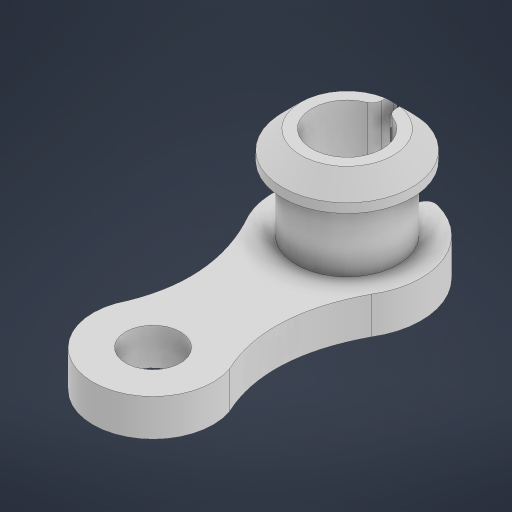
# Autodesk Inventor part: Servo_Pulley
Saved by Autodesk Inventor 2024 (Build 280153000, 153)
## iProperties
Created: 2025-09-10
Part Number: Servo_Pulley
Material: Generic
Document SubType Name: Modeling
Designer: kevin
Density: 1 g/cm^3
Appearance: Default
Author: kevin
Autodesk Inventor part; units mm, degrees
ref_plane "YZ Plane" through (0, 0, 0) normal (1, 0, 0) x (0, 1, 0)
ref_plane "XZ Plane" through (0, 0, 0) normal (0, 1, 0) x (-1, 0, 0)
ref_plane "XY Plane" through (0, 0, 0) normal (0, 0, 1) x (1, 0, 0)
sketch "Sketch1" plane through (0, 0, 0) normal (0, 1, 0) x (-1, 0, 0)
  circle A0 centre (0, 0) radius 2.95
  circle A1 centre (0, 0) radius 6.5
  circle A2 centre (0, -21) radius 8
  spline S0 degree 2 poles (6.1434, -2.1233) (2.6668, -9.5534) (7.2026, -17.5183) knots 0 0 0 1 1 1
  line L0 (0, 0) -> (0, -21) construction
  spline S1 degree 2 poles (-6.1434, -2.1233) (-2.6668, -9.5534) (-7.2026, -17.5183) knots 0 0 0 1 1 1
  point P0 (4.6554, -9.4486)
  point P1 (-4.6554, -9.4486)
  point P2 (-6.1434, -2.1233)
  point P3 (-6.812, -16.8052)
  dimension "d1" = 13
  dimension "d2" = 16
  dimension "d0" = 5.9
  dimension "d3" = 21
  constraints: 3 symmetric about line, 2 coincident, 2 end point, 1 centre point, 1 vertical, 12 other
  measures "d0" diameter of A0
  measures "d3" distance of L0.end point (0, 0)
extrude "Extrusion1" add sketch "Sketch1" along normal blind 4 contours A1 S0 S1 | A1 S0 A2 S1 | S1 A2 | A2 S0 S1
sketch "Sketch2" plane through (0, 4, 0) normal (0, 1, 0) x (1, 0, 0)
  arc A0 (6.812, 16.8052) -> (-7.2026, 17.5183) centre (0, 21) ccw projected
  arc A1 (-6.1434, 2.1233) -> (6.1434, 2.1233) centre (0, 0) ccw projected
  circle A2 centre (0, 0) radius 2.95 projected
  circle A3 centre (0, 21) radius 5.5
  line L0 (0.75, 12.2819) -> (-0.75, 12.2819)
  line L1 (-0.75, 12.2819) -> (-0.75, 29.7181)
  line L2 (-0.75, 29.7181) -> (0.75, 29.7181)
  line L3 (0.75, 29.7181) -> (0.75, 12.2819)
  line L4 (0.75, 12.2819) -> (-0.75, 29.7181) construction
  line L5 (-0.75, 12.2819) -> (0.75, 29.7181) construction
  circle A4 centre (0, 21) radius 3.8038
  point P0 (0.75, 26.4486)
  point P1 (0.75, 15.5514)
  point P2 (-0.75, 15.5514)
  point P3 (-0.75, 26.4486)
  point P4 (-0.75, 24.7291)
  point P5 (0.75, 24.7291)
  dimension "d6" = 11
  dimension "d7" = 1.5
  constraints: 12 end point, 2 centre point, 2 coincident, 2 midpoint, 2 parallel, 1 horizontal, 1 perpendicular, 2 other
  measures "d6" diameter of A3
  measures "d7" distance of L1.end L2.end
extrude "Extrusion2" cut sketch "Sketch2" against normal blind 5 contours L3 A3 L1 A0 | A0 L1 L2 L3 | L3 A4 L1 A3 | A4 L3 | L3 A4 L1 | L1 A4 picked at (-0.5838, 25.3244)
extrude "Extrusion3" add sketch "Sketch2" along normal blind 7 contours A3 L3 A4 | L1 A4 A3 | L1 A4 L3 A3 picked at (-0.5838, 16.6756)
sketch "Sketch4" plane through (0, 11, 0) normal (0, 1, 0) x (1, 0, 0)
  line L0 (-0.75, 24.7291) -> (-0.75, 26.4486) projected
  arc A0 (-0.75, 26.4486) -> (0.75, 26.4486) centre (0, 21) ccw projected
  line L1 (0.75, 26.4486) -> (0.75, 24.7291) projected
  arc A1 (-0.75, 24.7291) -> (0.75, 24.7291) centre (0, 21) ccw projected
  circle A2 centre (0, 21) radius 5.5 projected
  circle A3 centre (0, 21) radius 3.8038 projected
  circle A4 centre (0, 21) radius 7
  line L2 (-0.75, 12.2819) -> (-0.75, 29.7181) projected
  line L3 (0.75, 29.7181) -> (0.75, 12.2819) projected
  point P0 (0, 0)
  point P1 (0.75, 27.9597)
  point P2 (-0.75, 27.9597)
  dimension "d12" = 1.5
  constraints: 1 centre point
  measures "d12" radial gap between concentric circles of A2 A4
extrude "Extrusion4" add sketch "Sketch4" along normal blind 3 contours A1 L2 A0 L0 | A0 L2 A4 | A1 L3 A0 L2 | L1 A0 L3 A1 | A0 L3 A4 L2 | L3 A4 A0
chamfer "Chamfer1" distance 2 angle 45 1 edges at (0, 14, -14)
fillet "Fillet1" radius 1 8 edges at (0.75, 2, -28.9648) (-0.75, 2, -28.9648) (0.75, 12.5, -24.7291) (0.75, 2, -24.7291) (-0.75, 12.5, -24.7291) (-0.75, 2, -24.7291) (0.75, 11.5, -27.9597) (-0.75, 11.5, -27.9597)
body "Solid1"
